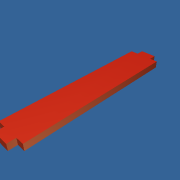
# Autodesk Inventor part: Acrylic_2.2_Lower
Saved by Autodesk Inventor 2012 (Build 160160000, 160)
## iProperties
Created: 2014-03-29
Part Number: Acrylic_2.2_Lower
Material: Default
Document SubType Name: Modeling
Designer: Admin
Density: 1 g/cm^3
Author: Admin
Autodesk Inventor part; units mm, degrees
ref_plane "YZ Plane" through (0, 0, 0) normal (1, 0, 0) x (0, 1, 0)
ref_plane "XZ Plane" through (0, 0, 0) normal (0, 1, 0) x (-1, 0, 0)
ref_plane "XY Plane" through (0, 0, 0) normal (0, 0, 1) x (1, 0, 0)
sketch "Sketch1" plane through (0, 0, 0) normal (0, 0, 1) x (1, 0, 0)
  line L0 (-7, 0) -> (7, 0) projected
  line L1 (0, -38.5) -> (0, 38.5) projected
  line L2 (5, 25) -> (5, -25)
  line L3 (-5, -25) -> (-5, 25)
  line L4 (-2.5, -25) -> (-2.5, -27.5)
  line L5 (-2.5, -27.5) -> (2.5, -27.5)
  line L6 (2.5, -27.5) -> (2.5, -25)
  line L7 (5, -25) -> (2.5, -25)
  line L8 (-2.5, -25) -> (-5, -25)
  line L9 (-2.5, 25) -> (-2.5, 27.5)
  line L10 (-2.5, 27.5) -> (2.5, 27.5)
  line L11 (2.5, 27.5) -> (2.5, 25)
  line L12 (-5, 25) -> (-2.5, 25)
  line L13 (2.5, 25) -> (5, 25)
  point P0 (0, 0)
  dimension "d0" = 10
  dimension "d1" = 50
  dimension "d3" = 5
  dimension "d7" = 2.5
  dimension "d8" = 2.5
  dimension "d10" = 2.5
  dimension "d11" = 2.5
  dimension "d12" = 2.5
  constraints: 24 end point, 9 perpendicular, 6 parallel, 2 horizontal
  measures "d0" distance of L2.end L3.start
  measures "d1" distance of L2.start L2.end
  measures "d3" distance between parallel lines of L2 L1
  measures "d7" distance between parallel lines of L1 L4
  measures "d8" distance between parallel lines of L6 L1
  measures "d10" distance between parallel lines of L1 L9
  measures "d11" distance between parallel lines of L11 L1
  measures "d12" distance between parallel lines of L7 L5
extrude "Extrusion1" add sketch "Sketch1" along normal blind 2.2
equation "\"d3\" = 0.5 * d0"
equation "\"d2\" = 0.5 * d1"
body "Solid1"
